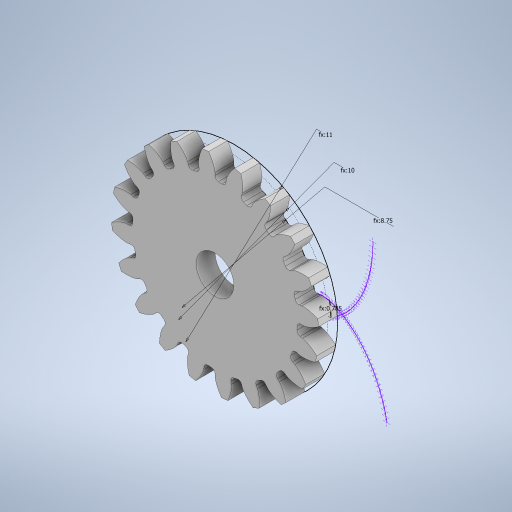
# Autodesk Inventor part: 齒輪
Saved by Autodesk Inventor 2024 (Build 280153000, 153)
## iProperties
Created: 2024-04-20
Part Number: 齒輪
Material: 一般
Document SubType Name: Modeling
Designer: rumse
Density: 1 g/cm^3
Appearance: 預設
Author: rumse
Autodesk Inventor part; units mm, degrees
note: some values were not read from the file. Left out: dimensions or parameters whose unit could not be read.
ref_plane "YZ Plane" through (0, 0, 0) normal (1, 0, 0) x (0, 1, 0)
ref_plane "XZ Plane" through (0, 0, 0) normal (0, 1, 0) x (-1, 0, 0)
ref_plane "XY Plane" through (0, 0, 0) normal (0, 0, 1) x (1, 0, 0)
sketch "草圖2" plane through (0, 0, 0) normal (0, 0, 1) x (1, 0, 0)
  circle A0 centre (0, 0) radius 4.375
  circle A1 centre (0, 0) radius 5 construction
  circle A2 centre (0, 0) radius 5.5
  spline S0 degree 4 poles (4.6985, 0) (4.7002, 0) (4.7088, 0.0003) (4.7231, 0.0015) (4.7472, 0.0045) (4.7725, 0.0086) (4.8034, 0.0147) (4.8396, 0.0232) (4.8811, 0.0344) (4.9276, 0.0487) (4.979, 0.0664) (5.0351, 0.0881) (5.0957, 0.1139) (5.1605, 0.1442) (5.2294, 0.1794) (5.3019, 0.2197) (5.378, 0.2655) (5.4572, 0.317) (5.5392, 0.3745) (5.6238, 0.4383) (5.7105, 0.5087) (5.799, 0.5857) (5.889, 0.6698) (5.9801, 0.7609) (6.0718, 0.8594) (6.1638, 0.9653) (6.2556, 1.0788) (6.3468, 1.2001) (6.4371, 1.3291) (6.5259, 1.466) (6.6128, 1.6108) (6.6974, 1.7636) (6.7793, 1.9244) (6.8578, 2.0931) (6.9327, 2.2697) (7.0034, 2.4541) (7.0695, 2.6464) (7.1306, 2.8463) (7.1861, 3.0537) (7.2356, 3.2685) (7.2787, 3.4905) (7.3149, 3.7196) (7.3549, 4.0464) (7.374, 4.3217) (7.3803, 4.5402) (7.3803, 4.6985) knots 0 0 0 0 0 0.014326 0.022769 0.032603 0.043639 0.055754 0.068854 0.08287 0.097744 0.113428 0.129883 0.147072 0.164967 0.183539 0.202765 0.222623 0.243094 0.26416 0.285804 0.308011 0.330767 0.35406 0.377877 0.402206 0.427038 0.452362 0.478169 0.50445 0.531197 0.558401 0.586055 0.614151 0.642684 0.671646 0.701031 0.730833 0.761047 0.791666 0.822685 0.8541 0.885905 0.918096 1 1 1 1 1
  line L0 (4.6985, 0) -> (4.375, 0)
  arc A3 (4.9994, 0.0745) -> (4.9262, 0.8557) centre (0, 0) ccw
  line L1 (4.9782, 0.4665) -> (0, 0)
  spline S1 degree 4 poles (4.6166, 0.873) (4.6184, 0.8733) (4.6268, 0.8746) (4.6412, 0.8761) (4.6654, 0.8776) (4.691, 0.8783) (4.7225, 0.878) (4.7597, 0.8765) (4.8025, 0.8732) (4.8508, 0.8677) (4.9047, 0.8598) (4.9638, 0.849) (5.0281, 0.8349) (5.0975, 0.8172) (5.1716, 0.7954) (5.2504, 0.7693) (5.3337, 0.7384) (5.421, 0.7025) (5.5123, 0.6612) (5.6073, 0.6142) (5.7056, 0.5612) (5.8069, 0.5019) (5.9109, 0.4361) (6.0173, 0.3635) (6.1257, 0.2837) (6.2358, 0.1967) (6.3471, 0.1023) (6.4593, 0.0001) (6.572, -0.1099) (6.6847, -0.228) (6.797, -0.3541) (6.9085, -0.4885) (7.0188, -0.6313) (7.1273, -0.7824) (7.2337, -0.942) (7.3375, -1.1101) (7.4381, -1.2867) (7.5352, -1.4718) (7.6283, -1.6653) (7.7169, -1.8672) (7.8005, -2.0774) (7.8786, -2.2957) (7.9786, -2.6094) (8.0486, -2.8763) (8.0954, -3.0898) (8.1248, -3.2454) knots 0 0 0 0 0 0.014326 0.022769 0.032603 0.043639 0.055754 0.068854 0.08287 0.097744 0.113428 0.129883 0.147072 0.164967 0.183539 0.202765 0.222623 0.243094 0.26416 0.285804 0.308011 0.330767 0.35406 0.377877 0.402206 0.427038 0.452362 0.478169 0.50445 0.531197 0.558401 0.586055 0.614151 0.642684 0.671646 0.701031 0.730833 0.761047 0.791666 0.822685 0.8541 0.885905 0.918096 1 1 1 1 1
  line L2 (4.6166, 0.873) -> (4.2988, 0.8129)
  point P0 (4.7013, 0.0001)
  point P1 (4.7099, 0.0005)
  point P2 (4.7242, 0.0018)
  point P3 (4.744, 0.0043)
  point P4 (4.7695, 0.0083)
  point P5 (4.8004, 0.0143)
  point P6 (4.8366, 0.0227)
  point P7 (4.8781, 0.0338)
  point P8 (4.9246, 0.0481)
  point P9 (4.976, 0.0658)
  point P10 (5.0322, 0.0874)
  point P11 (5.0928, 0.1131)
  point P12 (5.1576, 0.1434)
  point P13 (5.2265, 0.1785)
  point P14 (5.299, 0.2187)
  point P15 (5.3751, 0.2644)
  point P16 (5.4543, 0.3159)
  point P17 (5.5364, 0.3734)
  point P18 (5.6209, 0.4371)
  point P19 (5.7077, 0.5074)
  point P20 (5.7962, 0.5844)
  point P21 (5.8862, 0.6683)
  point P22 (5.9773, 0.7594)
  point P23 (6.069, 0.8578)
  point P24 (6.161, 0.9637)
  point P25 (6.2529, 1.0771)
  point P26 (6.3442, 1.1983)
  point P27 (6.4345, 1.3273)
  point P28 (6.5233, 1.4641)
  point P29 (6.6103, 1.6089)
  point P30 (6.6949, 1.7616)
  point P31 (6.7768, 1.9223)
  point P32 (6.8554, 2.0909)
  point P33 (6.9303, 2.2674)
  point P34 (7.001, 2.4518)
  point P35 (7.0672, 2.644)
  point P36 (7.1283, 2.8438)
  point P37 (7.1838, 3.0512)
  point P38 (7.2334, 3.2659)
  point P39 (7.2765, 3.4879)
  point P40 (7.3128, 3.7169)
  point P41 (7.3417, 3.9527)
  point P42 (7.3629, 4.1951)
  point P43 (7.3759, 4.4438)
  point P44 (4.6195, 0.8735)
  point P45 (4.628, 0.8746)
  point P46 (4.6422, 0.876)
  point P47 (4.6622, 0.8773)
  point P48 (4.688, 0.878)
  point P49 (4.7195, 0.8778)
  point P50 (4.7566, 0.8763)
  point P51 (4.7995, 0.8731)
  point P52 (4.8478, 0.8678)
  point P53 (4.9016, 0.8599)
  point P54 (4.9608, 0.8491)
  point P55 (5.0251, 0.8351)
  point P56 (5.0944, 0.8174)
  point P57 (5.1686, 0.7957)
  point P58 (5.2474, 0.7697)
  point P59 (5.3306, 0.7389)
  point P60 (5.418, 0.703)
  point P61 (5.5093, 0.6618)
  point P62 (5.6043, 0.6149)
  point P63 (5.7026, 0.562)
  point P64 (5.8039, 0.5027)
  point P65 (5.9079, 0.437)
  point P66 (6.0143, 0.3644)
  point P67 (6.1227, 0.2848)
  point P68 (6.2328, 0.1978)
  point P69 (6.3441, 0.1034)
  point P70 (6.4564, 0.0013)
  point P71 (6.569, -0.1086)
  point P72 (6.6817, -0.2266)
  point P73 (6.7941, -0.3527)
  point P74 (6.9056, -0.487)
  point P75 (7.0159, -0.6297)
  point P76 (7.1245, -0.7808)
  point P77 (7.2309, -0.9403)
  point P78 (7.3347, -1.1083)
  point P79 (7.4354, -1.2848)
  point P80 (7.5325, -1.4698)
  point P81 (7.6256, -1.6633)
  point P82 (7.7142, -1.8651)
  point P83 (7.7979, -2.0752)
  point P84 (7.876, -2.2934)
  point P85 (7.9483, -2.5198)
  point P86 (8.0141, -2.754)
  point P87 (8.0731, -2.9959)
  point P88 (5.4895, 0.34)
  point P89 (5.4571, 0.6859)
  dimension "d3" = 8.75
  dimension "d4" = 11
  dimension "d5" = 10
  dimension "d12" = 0.7854
  constraints: 47 symmetric about line, 6 end point, 5 point on circle, 3 centre point, 3 coincident, 2 horizontal, 1 concentric, 96 other
  measures "d4" diameter of A2
  measures "d5" diameter of A1
extrude "擠出1" add sketch "草圖2" along normal blind 1 contours A0 | L2 S1 A3 L1 A0 | A0 L1 A3 S0 L0 | A3 S1 A2 S0
fillet "圓角1" radius 0.19 2 edges at (4.2988, 0.8129, 0.5) (4.375, 0, 0.5)
pattern_circular "環形陣列1" count 20 over 360 about axis through (0, 0, 0) along (0, 0, 1) of "擠出1", "圓角1"
sketch "草圖4" plane through (0, 0, 1) normal (0, 0, 1) x (1, 0, 0)
  point P0 (0, 0)
hole "孔1" at (0, 0, 1) direction (0, 0, -1) diameter 2 end through all
equation "\"d3\" = dedendum_diameter"
equation "\"d4\" = addendum_diameter"
equation "\"d5\" = pitch_diameter"
equation "\"d12\" = tooth_thickness"
equation "\"d15\" = fillet_radius"
equation "\"whole_depth\" = 2.25 * module"
equation "\"tooth_thickness\" = 1.5708 * module"
equation "\"circular_pitch\" = 3.14159 * module"
equation "\"addendum\" = module"
equation "\"dedendum\" = 1.25 * module"
equation "\"addendum_diameter\" = pitch_diameter + 2 * addendum"
equation "\"dedendum_diameter\" = pitch_diameter - 2 * dedendum"
equation "\"pressure_angle\" = 20deg"
equation "\"fillet_radius\" = 0.38 * module"
equation "\"rack_dedendum\" = 0.25 * module"
equation "\"pitch_diameter\" = 10"
